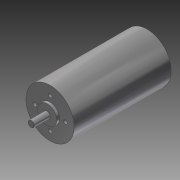
# Autodesk Inventor part: Moteur Crouzet
Saved by Autodesk Inventor 2016 SP1 (Build 200210100, 210)
## iProperties
Created: 2015-09-22
Part Number: Moteur Crouzet
Material: Acier inoxydable
Document SubType Name: Modeling
Designer: sd
Density: 8.08 g/cm^3
Appearance: Semi-poli
Mass: 3221.22 g
Surface Area: 334.531 cm^2
Volume: 398.666 cm^3
Author: sd
Autodesk Inventor part; units mm, degrees
ref_plane "YZ Plane" through (0, 0, 0) normal (1, 0, 0) x (0, 1, 0)
ref_plane "XZ Plane" through (0, 0, 0) normal (0, 1, 0) x (-1, 0, 0)
ref_plane "XY Plane" through (0, 0, 0) normal (0, 0, 1) x (1, 0, 0)
sketch "Esquisse1" plane through (0, 0, 0) normal (0, 1, 0) x (-1, 0, 0)
  circle A0 centre (0, 0) radius 31.5
  dimension "d0" = 63
  constraints: 1 centre point, 1 coincident
  measures "d0" diameter of A0
extrude "Extrusion1" add sketch "Esquisse1" along normal blind 127
sketch "Esquisse2" plane through (0, 127, 0) normal (0, 1, 0) x (1, 0, 0)
  circle A0 centre (0, 0) radius 31.5 projected
  circle A1 centre (0, 0) radius 12.5
  dimension "d3" = 25
  constraints: 1 centre point, 1 coincident
  measures "d3" diameter of A1
extrude "Extrusion2" add sketch "Esquisse2" along normal blind 2.5 contours A1
sketch "Esquisse3" plane through (0, 0, 0) normal (0, -1, 0) x (1, 0, 0)
  circle A0 centre (0, 0) radius 31.5 projected
  circle A1 centre (0, 0) radius 12.5
  dimension "d6" = 25
  constraints: 1 centre point, 1 coincident
  measures "d6" diameter of A1
extrude "Extrusion3" add sketch "Esquisse3" along normal blind 3.7 contours A1
sketch "Esquisse4" plane through (0, -3.7, 0) normal (0, -1, 0) x (1, 0, 0)
  circle A0 centre (0, 0) radius 12.5 projected
  circle A1 centre (0, 0) radius 4
  dimension "d9" = 8
  constraints: 1 centre point, 1 coincident
  measures "d9" diameter of A1
extrude "Extrusion4" add sketch "Esquisse4" along normal blind 21.3 contours A1
chamfer "Chanfrein1" distance 0.5 angle 45 1 edges at (-4, -25, 0)
sketch "Esquisse5" plane through (0, 0, 0) normal (0, -1, 0) x (1, 0, 0)
  circle A0 centre (0, 0) radius 12.5 projected
  circle A1 centre (0, 20) radius 2.5
  dimension "d15" = 5
  dimension "d16" = 20
  constraints: 1 centre point
  measures "d15" diameter of A1
  measures "d16" distance of A0.centre A1.centre
extrude "Extrusion5" cut sketch "Esquisse5" against normal blind 10 contours A1
pattern_circular "Réseau circulaire1" count 4 over 360 about axis through (0, -3.7, 0) along (0, -1, 0) of "Extrusion5"
sketch "Esquisse6" plane through (0, 127, 0) normal (0, 1, 0) x (1, 0, 0)
  circle A0 centre (0, 0) radius 12.5 projected
  circle A1 centre (0, 20) radius 2.5
  dimension "d22" = 5
  dimension "d23" = 20
  constraints: 1 centre point
  measures "d22" diameter of A1
  measures "d23" distance of A0.centre A1.centre
extrude "Extrusion6" cut sketch "Esquisse6" against normal blind 7 contours A1
pattern_circular "Réseau circulaire2" count 4 over 360 about axis through (0, 127, 0) along (0, 1, 0) of "Extrusion6"
